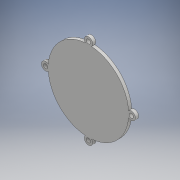
# Autodesk Inventor part: tapaRGB-anillo
Saved by Autodesk Inventor 2018 (Build 220112000, 112)
## iProperties
Created: 2019-01-29
Part Number: tapaRGB-anillo
Material: Generic
Document SubType Name: Modeling
Designer: Estudiante
Density: 1 g/cm^3
Appearance: Default
Author: Estudiante
Autodesk Inventor part; units mm, degrees
ref_plane "YZ Plane" through (0, 0, 0) normal (1, 0, 0) x (0, 1, 0)
ref_plane "XZ Plane" through (0, 0, 0) normal (0, 1, 0) x (-1, 0, 0)
ref_plane "XY Plane" through (0, 0, 0) normal (0, 0, 1) x (1, 0, 0)
sketch "Sketch1" plane through (0, 0, 0) normal (0, 1, 0) x (-1, 0, 0)
  arc A0 (-1.5117, -19.1905) -> (1.5117, -19.1905) centre (0, -20.5) ccw
  circle A1 centre (0, 20.5) radius 1
  circle A2 centre (0, -20.5) radius 1
  arc A3 (-1.5117, 19.1905) -> (-19.1905, 1.5118) centre (0, 0) ccw
  arc A4 (-19.1905, 1.5118) -> (-19.1905, -1.5118) centre (-20.4999, 0) ccw
  arc A5 (-19.1905, -1.5118) -> (-1.5117, -19.1905) centre (0, 0) ccw
  arc A6 (-1.5117, -19.1905) -> (1.5117, -19.1905) centre (0, -20.5) ccw
  arc A7 (1.5117, -19.1905) -> (19.1909, -1.5076) centre (0, 0) ccw
  arc A8 (19.1909, -1.5076) -> (19.1909, 1.5076) centre (20.505, 0) ccw
  arc A9 (19.1909, 1.5076) -> (1.5117, 19.1905) centre (0, 0) ccw
  arc A10 (1.5117, 19.1905) -> (-1.5117, 19.1905) centre (0, 20.5) ccw
  circle A11 centre (-20.4999, 0) radius 1
  arc A12 (-18.5, -0.0197) -> (-18.5, 0.0197) centre (-20.4999, 0) ccw
  circle A13 centre (20.505, 0) radius 1
  constraints: 20 point on circle, 14 centre point
extrude "Extrusion1" add sketch "Sketch1" along normal blind 1.5
body "Solid1"
